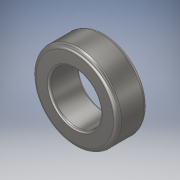
# Autodesk Inventor part: U51105
Saved by Autodesk Inventor 2017 SP1 (Build 210196100, 196)
## iProperties
Created: 2017-06-04
Part Number: U51105
Material: Steel, Carbon
Catalog Web Link: https://www.amazon.com/uxcell-51105-Axial-Thrust-Bearings/dp/B008VOZ83G/ref=sr_1_10?ie=UTF8&qid=1496590275&sr=8-10&keywords=thrust+bearings+25+mm
Document SubType Name: Modeling
Designer: Zach
Density: 7.85 g/cm^3
Appearance: Semi-Polished
Author: Zach
Autodesk Inventor part; units mm, degrees
ref_plane "YZ Plane" through (0, 0, 0) normal (1, 0, 0) x (0, 1, 0)
ref_plane "XZ Plane" through (0, 0, 0) normal (0, 1, 0) x (-1, 0, 0)
ref_plane "XY Plane" through (0, 0, 0) normal (0, 0, 1) x (1, 0, 0)
sketch "Sketch1" plane through (0, 0, 0) normal (0, 0, 1) x (1, 0, 0)
  circle A0 centre (0, 0) radius 12.5
  circle A1 centre (0, 0) radius 21
  dimension "d0" = 25
  dimension "d1" = 42
  constraints: 2 centre point, 2 coincident
  measures "d0" diameter of A0
  measures "d1" diameter of A1
extrude "Extrusion1" add sketch "Sketch1" along normal blind 15
fillet "Fillet1" radius 2 2 edges at (-21, 0, 15) (-21, 0, 0)
fillet "Fillet2" radius 1 2 edges at (-12.5, 0, 0) (-12.5, 0, 15)
body "Solid1"
